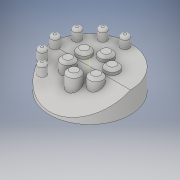
# Autodesk Inventor part: 示範一
Saved by Autodesk Inventor 2017 (Build 210142000, 142)
## iProperties
Part Number: 示範一
Material: 一般
Document SubType Name: Modeling
Designer: user
Density: 1 g/cm^3
Appearance: 預設
Author: user
Autodesk Inventor part; units mm, degrees
ref_plane "YZ Plane" through (0, 0, 0) normal (1, 0, 0) x (0, 1, 0)
ref_plane "XZ Plane" through (0, 0, 0) normal (0, 1, 0) x (-1, 0, 0)
ref_plane "XY Plane" through (0, 0, 0) normal (0, 0, 1) x (1, 0, 0)
sketch "草圖1" plane through (0, 0, 0) normal (0, 1, 0) x (-1, 0, 0)
  circle A0 centre (0, 0) radius 15
  dimension "d0" = 30
  constraints: 1 centre point, 1 coincident
  measures "d0" diameter of A0
extrude "擠出1" add sketch "草圖1" along normal blind 8
sketch "草圖3" plane through (0, 0, 0) normal (1, 0, 0) x (0, 1, 0)
  line L0 (0, 15) -> (8, 15) projected
  line L1 (1, 15) -> (8, 0)
  line L2 (8, -15) -> (8, 15) projected
  line L3 (8, 0) -> (8, 15)
  line L4 (8, 15) -> (1, 15)
  line L5 (0, 15) -> (0, -15) projected
  point P0 (0, 0)
  dimension "d3" = 1
  constraints: 6 end point, 1 midpoint, 1 perpendicular, 1 point on line, 1 vertical
  measures "d3" distance from line of L1.start L5
extrude "擠出2" cut sketch "草圖3" along normal mid plane 300
sketch "草圖4" plane through (0, 8, 0) normal (0, 1, 0) x (1, 0, 0)
  circle A0 centre (0, 0) radius 6 construction
  circle A1 centre (0, 6) radius 2.5
  line L0 (0, 0) -> (0, 9.7931)
  line L1 (-3.2998, 6) -> (3.1702, 6)
  dimension "d6" = 12
  dimension "d7" = 5
  constraints: 2 vertical alignment, 1 centre point, 1 coincident, 8 other
  measures "d7" diameter of A1
extrude "擠出3" add sketch "草圖4" along normal blind 2
chamfer "倒角1" distance 1 angle 45 1 edges at (-2.5, 10, -6) measured on face at (1.1976, 10, -6.694)
pattern_circular "環形陣列1" count 6 over 360 about axis through (0, 0, 0) along (0, -1, 0) of "擠出3", "倒角1"
sketch "草圖6" plane through (-5.1962, 8, 3) normal (0, -1, 0) x (1, 0, 0)
  circle A0 centre (0, 0) radius 2.5
  point P0 (5.1962, -3)
  dimension "d18" = 5
  constraints: 1 centre point
  measures "d18" diameter of A0
extrude "擠出5" add sketch "草圖6" along normal up to next
sketch "草圖8" plane through (0, 8, 6) normal (0, -1, 0) x (1, 0, 0)
  circle A0 centre (0, 0) radius 2.5
  point P0 (0, -6)
  constraints: 1 centre point
extrude "擠出6" add sketch "草圖8" along normal up to next
sketch "草圖9" plane through (5.1962, 8, 3) normal (0, -1, 0) x (1, 0, 0)
  circle A0 centre (0, 0) radius 2.5
  point P0 (-5.1962, -3)
  constraints: 1 centre point
extrude "擠出7" add sketch "草圖9" along normal up to next
sketch "草圖10" plane through (0, 8, 0) normal (0, 1, 0) x (1, 0, 0)
  circle A0 centre (0, 0) radius 13
  circle A1 centre (0, 13) radius 1.5
  line L0 (0, 13.5724) -> (0, 0)
  dimension "d25" = 26
  dimension "d26" = 3
  constraints: 2 coincident, 2 end point, 1 centre point, 1 point on line, 1 vertical, 1 vertical alignment, 2 other
  measures "d26" diameter of A1
extrude "擠出8" add sketch "草圖10" along normal blind 4 contours A1 L0 A0 | A0 A1 | A0 L0 A1 picked at (0.3336, 13.4681)
fillet "圓角1" radius 1 1 edges at (-1.5, 12, -13)
pattern_circular "環形陣列2" count 6 over 150 about axis through (0, 0, 0) along (0, 1, 0) of "圓角1", "擠出8"
